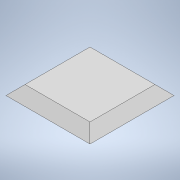
# Autodesk Inventor part: reed-switch-cap
Saved by Autodesk Inventor 2021 (Build 250183000, 183)
## iProperties
Created: 2021-01-14
Part Number: reed-switch-cap
Material: Generic
Document SubType Name: Modeling
Designer: Luke Kamols
Density: 1 g/cm^3
Appearance: Default
Author: Luke Kamols
Autodesk Inventor part; units mm, degrees
ref_plane "YZ Plane" through (0, 0, 0) normal (1, 0, 0) x (0, 1, 0)
ref_plane "XZ Plane" through (0, 0, 0) normal (0, 1, 0) x (-1, 0, 0)
ref_plane "XY Plane" through (0, 0, 0) normal (0, 0, 1) x (1, 0, 0)
sketch "Sketch1" plane through (0, 0, 0) normal (0, 1, 0) x (-1, 0, 0)
  line L0 (0, 0) -> (13.2, 0)
  line L1 (13.2, 0) -> (13.2, -13.2)
  line L2 (13.2, -13.2) -> (0, -13.2)
  line L3 (0, -13.2) -> (0, 0)
  dimension "d0" = 13.2
  dimension "d1" = 13.2
  constraints: 8 end point, 2 parallel, 1 horizontal, 1 perpendicular
  measures "d0" distance of L1.end L2.end
  measures "d1" distance of L0.end L1.end
extrude "Extrusion1" add sketch "Sketch1" along normal blind 1.5
chamfer "Chamfer1" distance 1.5 angle 45 4 edges at (0, 1.5, -6.6) (-6.6, 1.5, 0) (-13.2, 1.5, -6.6) (-6.6, 1.5, -13.2)
body "Solid1"
